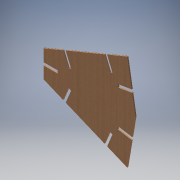
# Autodesk Inventor part: internalSupportBottom2
Saved by Autodesk Inventor 2019 (Build 230136000, 136)
## iProperties
Created: 2019-01-08
Part Number: internalSupportBottom2
Material: Wood (Cherry)
Document SubType Name: Modeling
Designer: gaincarlo
Density: 0.63 g/cm^3
Appearance: Cherry - Natural Low Gloss
Author: gaincarlo
Autodesk Inventor part; units mm, degrees
ref_plane "YZ Plane" through (0, 0, 0) normal (1, 0, 0) x (0, 1, 0)
ref_plane "XZ Plane" through (0, 0, 0) normal (0, 1, 0) x (-1, 0, 0)
ref_plane "Work Plane1" through (0, 0, -3) normal (0, 0, -1) x (-1, 0, 0)
sketch "Sketch1" plane through (0, 0, -3) normal (0, 0, -1) x (-1, 0, 0)
  line L0 (188.08, 47.916) -> (188.08, -47.916) projected
  line L1 (-110.3592, 171.5336) -> (188.08, 47.916) projected
  spline S0 degree 3 poles (-139.4832, 0) (-137.0244, 14.4817) (-134.5656, 28.9634) (-129.6218, 58.0812) (-127.1368, 72.7174) (-124.6518, 87.3535) (-122.1668, 101.99) (-119.6817, 116.6264) (-114.9175, 144.6864) (-112.6384, 158.11) (-110.3592, 171.5336) knots 0.047 0.047 0.047 0.047 4.453683 4.453683 8.907367 8.907367 8.907367 13.361137 13.361137 17.44584 17.44584 17.44584 17.44584 projected
  spline S1 degree 3 poles (-110.3592, -171.5336) (-112.6384, -158.11) (-114.9175, -144.6864) (-119.6817, -116.6264) (-122.1668, -101.99) (-124.6518, -87.3535) (-127.1368, -72.7174) (-129.6218, -58.0812) (-134.5656, -28.9634) (-137.0244, -14.4817) (-139.4832, 0) knots 0.369067 0.369067 0.369067 0.369067 4.45377 4.45377 8.90754 8.90754 8.90754 13.361224 13.361224 17.767907 17.767907 17.767907 17.767907 projected
  line L2 (188.08, -47.916) -> (-110.3592, -171.5336) projected
  point P0 (0, 0)
extrude "Extrusion1" add sketch "Sketch1" along normal blind 4
sketch "Sketch2" plane through (0, 0, -7) normal (0, 0, -1) x (-1, 0, 0)
  line L0 (188.08, -47.916) -> (188.08, 47.916) construction
  line L1 (188.08, 47.916) -> (-110.3592, 171.5336) construction
  line L2 (-110.3592, -171.5336) -> (188.08, -47.916) construction
  line L3 (138.08, 5) -> (188.08, 5)
  line L4 (188.08, 5) -> (188.08, -5)
  line L5 (188.08, -5) -> (138.08, -5)
  line L6 (138.08, -5) -> (138.08, 5)
  line L7 (99.2388, -30.5956) -> (90, -34.4224)
  line L8 (90, -34.4224) -> (109.1342, -80.6164)
  line L9 (109.1342, -80.6164) -> (118.373, -76.7896)
  line L10 (118.373, -76.7896) -> (99.2388, -30.5956)
  line L11 (-48.5819, -91.8249) -> (-57.8207, -95.6518)
  line L12 (-57.8207, -95.6518) -> (-38.6866, -141.8457)
  line L13 (-38.6866, -141.8457) -> (-29.4478, -138.0189)
  line L14 (-29.4478, -138.0189) -> (-48.5819, -91.8249)
  line L15 (-78.5805, -60) -> (-127.875, -68.3695)
  line L16 (-127.875, -68.3695) -> (-126.2011, -78.2284)
  line L17 (-126.2011, -78.2284) -> (-76.9066, -69.8589)
  line L18 (-76.9066, -69.8589) -> (-78.5805, -60)
  line L19 (-76.9066, 69.8589) -> (-126.2011, 78.2284)
  line L20 (-126.2011, 78.2284) -> (-127.875, 68.3695)
  line L21 (-127.875, 68.3695) -> (-78.5805, 60)
  line L22 (-78.5805, 60) -> (-76.9066, 69.8589)
  line L23 (109.1342, 80.6164) -> (118.373, 76.7896)
  line L24 (118.373, 76.7896) -> (99.2388, 30.5956)
  line L25 (99.2388, 30.5956) -> (90, 34.4224)
  line L26 (90, 34.4224) -> (109.1342, 80.6164)
  line L27 (188.08, -47.916) -> (188.08, 47.916) projected
  line L28 (-110.3592, -171.5336) -> (188.08, -47.916) projected
  line L29 (188.08, 47.916) -> (-110.3592, 171.5336) projected
  line L30 (-29.4478, 138.0189) -> (-38.6866, 141.8457)
  line L31 (-38.6866, 141.8457) -> (-57.8207, 95.6518)
  line L32 (-57.8207, 95.6518) -> (-48.5819, 91.8249)
  line L33 (-48.5819, 91.8249) -> (-29.4478, 138.0189)
  point P0 (0, 0)
  point P1 (-139.4832, 0)
  point P2 (188.08, 0)
  dimension "d2" = 10
  dimension "d3" = 10
  dimension "d5" = 10
  dimension "d6" = 10
  dimension "d7" = 10
  dimension "d8" = 10
  dimension "d10" = 50
  dimension "d11" = 50
  dimension "d12" = 50
  dimension "d13" = 50
  dimension "d14" = 50
  dimension "d15" = 50
  dimension "d18" = 150
  dimension "d19" = 60
  dimension "d20" = 60
  dimension "d21" = 90
  dimension "d22" = 90
  dimension "d23" = 10
  dimension "d24" = 50
  dimension "d25" = 150
  constraints: 56 end point, 14 parallel, 11 perpendicular, 4 point on line, 2 midpoint, 1 collinear, 1 horizontal, 8 other
  measures "d2" distance of L23.start L23.end
  measures "d3" distance of L3.end L4.end
  measures "d5" distance of L8.end L9.end
  measures "d6" distance of L12.end L13.end
  measures "d7" distance of L19.end L20.end
  measures "d8" distance of L15.end L16.end
  measures "d10" distance of L25.end L23.start
  measures "d11" distance of L4.end L5.end
  measures "d12" distance of L9.end L7.start
  measures "d13" distance of L13.end L11.start
  measures "d14" distance of L16.end L17.end
  measures "d15" distance of L20.end L21.end
  measures "d18" distance between parallel lines of L14 L8
  measures "d19" vertical distance of L21.end point (0, 0)
  measures "d20" vertical distance of L15.start point (0, 0)
  measures "d21" horizontal distance of L25.end point (0, 0)
  measures "d22" horizontal distance of point (0, 0) L7.end
  measures "d23" distance of L32.end L31.end
  measures "d24" distance of L31.end L30.end
  measures "d25" distance between parallel lines of L33 L26
extrude "Extrusion2" cut sketch "Sketch2" against normal through all
body "Solid1"
